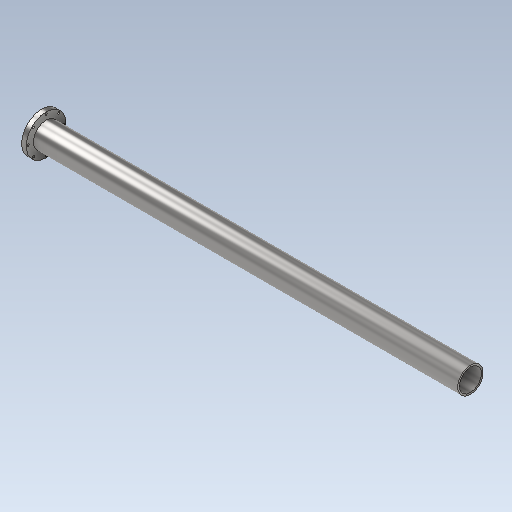
# Autodesk Inventor part: Lift.02.00.00.01
Saved by Autodesk Inventor 2021 (Build 250183000, 183)
## iProperties
Created: 2020-09-20
Part Number: Lift.02.00.00.01
Material: Сталь нержавеющая, 440C
Document SubType Name: Modeling
Designer: Kostya
Density: 7.75 g/cm^3
Appearance: С умеренной полировкой
Author: Kostya
Autodesk Inventor part; units mm, degrees
ref_plane "YZ Plane" through (0, 0, 0) normal (1, 0, 0) x (0, 1, 0)
ref_plane "XZ Plane" through (0, 0, 0) normal (0, 1, 0) x (-1, 0, 0)
ref_plane "XY Plane" through (0, 0, 0) normal (0, 0, 1) x (1, 0, 0)
sketch "Эскиз1" plane through (0, 0, 0) normal (0, 0, 1) x (1, 0, 0)
  line L0 (0, 0) -> (-3428.5795, 0)
  line L1 (-3285, 0) -> (-3285, 152.5)
  line L2 (-3285, 152.5) -> (-3250, 152.5)
  line L3 (-3250, 152.5) -> (-3250, 97.5)
  line L4 (-3250, 97.5) -> (0, 97.5)
  line L5 (0, 97.5) -> (0, 0)
  line L6 (0, 85) -> (-3250, 85)
  line L7 (-3250, 85) -> (-3250, 0)
  dimension "d0" = 3285
  dimension "d1" = 305
  dimension "d2" = 35
  dimension "d3" = 170
  dimension "d4" = 195
  constraints: 16 end point, 6 perpendicular, 3 point on line, 1 horizontal, 1 vertical, 1 vertical alignment
  measures "d0" distance between parallel lines of L5 L1
  measures "d1" diameter of L2 L0
  measures "d2" distance of L1.end L2.end
  measures "d3" diameter of L6 L0
  measures "d4" diameter of L4 L0
revolve "Вращение1" add sketch "Эскиз1" angle 360 about axis through (0, 0, 0) along (-1, 0, 0) contours L0 L1 L2 L3 L4 L5 L6 L7
sketch "Эскиз2" plane through (-3285, 0, 0) normal (-1, 0, 0) x (0, 0, 1)
  circle A0 centre (0, 0) radius 137.5 construction
  point P0 (0, 137.5)
  dimension "d6" = 275
  constraints: 2 vertical alignment, 1 coincident, 2 other
hole "Отверстие1" at (-3285, 137.5, 0) direction (1, 0, 0) diameter 17 end through all
pattern_circular "Круговой массив1" count 8 over 360 about axis through (-3267.5, 0, 0) along (1, 0, 0) of "Отверстие1"
